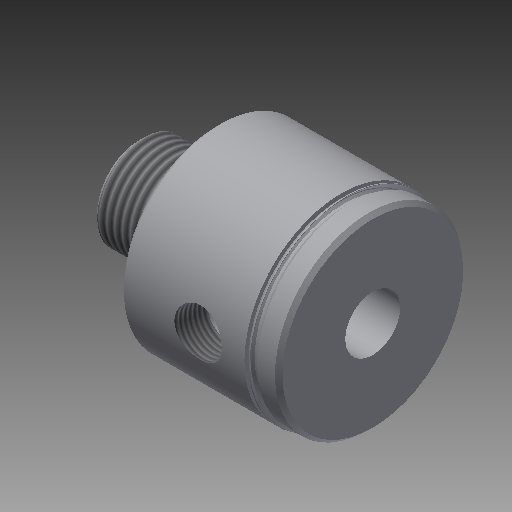
# Autodesk Inventor part: 17R000-0_rod_guide
Saved by Autodesk Inventor 2019.4 (Build 234330000, 330)
## iProperties
Category: PARTsolutions
Company: BIMBA
Created: 2020-02-18
Part Number: 17R000-0_rod_guide
Material: Generic
Catalog Web Link: www.cadenas.de
Description: Rod Guide-Original Line - Standard Air Cylinders
Vendor: BIMBA
Document SubType Name: Modeling
Designer: psadmin
Manufacturer: BIMBA
Mass: 37.006 g
Surface Area: 94.3607 cm^2
Volume: 37.006 cm^3
Density: 1 g/cm^3
Appearance: PSOLRGB-211-211-211
PSOL_IDENT_0: {$CADENAS_DATA\23d-libs\bimba\bimba_brand\bimba_imperial\bimba_full_line\original_line_cylinders\sta
PSOL_IDENT_1: ndard_air_cylinders\rod_guide.prj},251 {VTYP=3D},{NB=17R000-0_rod_guide},{LINA=17R000-0_rod_guide},{
PSOL_IDENT_2: NN=Rod Guide},{DATE=10.02.2020 11:55:59},{GEOMDATE=15.10.2019 12:06:01},{VERSION=},{LINEID=80},{WBVA
PSOL_IDENT_3: R=MNT,ACTING,NR,K,Q,T1,T2,T3,T4,MB,TRIM,CUSH,RODTRANS},{WBNUMERIC=MB,TRIM,CUSH,RODTRANS}  {NB=17R000
PSOL_IDENT_4: -0_rod_guide},{LINA=17R000-0_rod_guide},{KT=DUMMY},{PN=17R000},{BORE=1.50000000},{BOREPN=17},{MNT=},
PSOL_IDENT_5: {MNTALG='' , 'Front Nose' , 'BF' , 'Front Block' , 'BFT' , 'Front Trunnion' , 'A' , 'Adjustable Stro
PSOL_IDENT_6: ke','BR' , 'Rear Block'},{ACTING=R},{ACTINGALG= '' , 'Single Acting' , 'R' , 'Reverse/Double Acting'
PSOL_IDENT_7: },{NR=},{NRALG= '' , 'Without Non-rotating Rod' , 'NR' , 'With Non-rotating Rod' },{K=},{Q=},{QALG=
PSOL_IDENT_8: '' , 'Without Side Ported Rear Head' , 'Q' , 'With Side Ported Rear Head' },{T1=},{T2=},{T3=},{T4=}
PSOL_IDENT_9: ,{MB=0},{A1=1.8750},{A1N=1.3120},{A1P=1.8750},{A1B=2.3750},{A2=0.6250},{A2N=0.6250},{A2P=0.6250},{A3=
PSOL_IDENT_10: 1.0000},{A3N=0.1880},{A3P=1.0000},{A4=0.2525},{A4N=0.5000},{A4P=0.2525},{A5=0.0400},{A6=0.0000},{A6N=
PSOL_IDENT_11: 0.2500},{A6P=0.0000},{A7=0.2500},{A7N=0.6430},{A7P=0.2500},{A8=0.0300},{A8N=0.0300},{A8NR=0.0300},{D
PSOL_IDENT_12: 1=1.5565},{D1N=1.5565},{D1P=1.5565},{D1B=1.5800},{D2=1.5115},{D3=0.0000},{D3N=0.8120},{D3P=0.0000},{
PSOL_IDENT_13: D4=0.9690},{D4N=0.4730},{D4P=0.9690},{D4NR=0.4395},{D5=0.4420},{D5N=0.4420},{D5NR=0.4395},{C1=0.030}
PSOL_IDENT_14: ,{C2=0.0300},{C2N=0.0300},{C2P=0.0300},{C3=0.0000},{C3N=0.0000},{C3P=0.0000},{C4=0.0300},{C4N=0.0000
PSOL_IDENT_15: },{C4P=0.0300},{NDM=0.7500},{NDMN=0.7500},{NDMP=0.7500},{TAB=UNF},{D6=0.7475},{D6N=0.7475},{D6P=0.74
PSOL_IDENT_16: 75},{A9=0.0940},{A9N=0.0940},{A9P=0.0940},{D7=0.6535},{D7N=0.6535},{D7P=0.6535},{A10=0.0965},{A10N=0
PSOL_IDENT_17: .0965},{A10P=0.0965},{R1=0.0440},{R1N=0.0440},{R1P=0.0440},{D8=0.8120},{D9=0.7500},{D10=0.6880},{A11=
PSOL_IDENT_18: 0.8650},{A12=0.9590},{A13=1.1150},{A14=0.6250},{A14N=0.6250},{A14B=0.7190},{D11=0.2500},{D11N=0.2500
PSOL_IDENT_19: },{NDM2=0.4050},{NDM2N=0.4050},{NDM2DP=0.4200},{THREAD=0},{HEX=0.4375},{HEXN=0.4375},{S1=1.7500},{B1=
PSOL_IDENT_20: 0.1275},{B2=1.0050},{B22=0.0000},{DB=0.0000},{B3=0.6200},{B4=1.1300},{X1=0.1230},{X2=0.9975},{NDM3=0
PSOL_IDENT_21: .3125},{NDM4=0.2500},{NDM4DP=0.4950},{DD=1.7500},{CB=0.3750},{CBDP=0.2500},{PORT=1},{XT=1.0610},{XTX=
PSOL_IDENT_22: 1.0610},{XT1=0.5000},{XT2=0.3800},{NDMH=0.7500},{OD=1.5565},{ID=1.5115},{G=0.0000},{PNUT=0.5310},{TR
PSOL_IDENT_23: IM=0},{C11=0.3965},{C22=0.5625},{C33=0.3050},{C44=0.6250},{C55=0.8750},{CD1=0.2650},{CD2=0.1980},{CD
PSOL_IDENT_24: 3=0.1345},{CNDM3=0.2500},{CTAB3=UNS},{CUSH=0},{XX=1.13000},{LCD=0.0000},{RODTRANS=0.00000}
NN: Rod Guide
NT: Original Line - Standard Air Cylinders
NB: 17R000-0_rod_guide
NBSYN: $PN.-$RODTRANS._rod_guide
LINA: 17R000-0_rod_guide
BORE: 0
BOREPN: 17
MNT: Front Nose
MNTALG: '' , 'Front Nose' , 'BF' , 'Front Block' , 'BFT' , 'Front Trunnion' , 'A' , 'Adjustable Stroke','BR' , 'Rear Block'
ACTING: Reverse/Double Acting
NR: Without Non-rotating Rod
K: Standard
Q: Without Side Ported Rear Head
T1: without T1
T2: without T2
T3: without T3
T4: without T4
MB: 0
A1N: 1.312
A1P: 1.875
A1B: 2.375
A2N: 0.625
A2P: 0.625
A3N: 0.188
A3P: 1
A4N: 0.5
A4P: 0.2525
A5: 0.04
A6N: 0.25
A6P: 0
A7N: 0.643
A7P: 0.25
A8N: 0.03
A8NR: 0.03
D1N: 1.5565
D1P: 1.5565
D1B: 1.58
D2: 1.5115
D3N: 0.812
D3P: 0
D4N: 0.473
D4P: 0.969
D4NR: 0.4395
D5N: 0.442
D5NR: 0.4395
C1: 0.03
C2N: 0.03
C2P: 0.03
C3N: 0
C3P: 0
C4N: 0
C4P: 0.03
NDMN: 0.75
NDMP: 0.75
TAB: UNF
D6N: 0.7475
D6P: 0.7475
A9N: 0.094
A9P: 0.094
D7N: 0.6535
D7P: 0.6535
A10N: 0.0965
A10P: 0.0965
R1N: 0.044
R1P: 0.044
D8: 0.812
D9: 0.75
D10: 0.688
A11: 0.865
A12: 0.959
A13: 1.115
A14N: 0.625
A14B: 0.719
D11N: 0.25
NDM2N: 0.405
NDM2DP: 0.42
HEXN: 0.4375
S1: 1.75
B1: 0.1275
B2: 1.005
B22: 0
DB: 0
B3: 0.62
B4: 1.13
X1: 0.123
X2: 0.9975
NDM3: 0.3125
NDM4: 0.25
NDM4DP: 0.495
DD: 1.75
CB: 0.375
CBDP: 0.25
XTX: 1.061
XT1: 0.5
XT2: 0.38
NDMH: 0.75
TRIM: 0
C11: 0.3965
C22: 0.5625
C33: 0.305
C44: 0.625
C55: 0.875
CD1: 0.265
CD2: 0.198
CD3: 0.1345
CNDM3: 0.25
CTAB3: UNS
CUSH: 0
LCD: 0
RODTRANS: 0
SUPPLIER: BIMBA
ARTICLENO: 17R000-0_rod_guide
BOMINFO: 17R000-0_rod_guide
CREATOR: CADENAS GmbH
Title: 17R000-0_rod_guide
Author: Cadenas PARTsolutions
Comments: Original Line - Standard Air Cylinders
Autodesk Inventor part; units mm, degrees
ref_plane "YZ Plane" through (0, 0, 0) normal (1, 0, 0) x (0, 1, 0)
ref_plane "XZ Plane" through (0, 0, 0) normal (0, 1, 0) x (-1, 0, 0)
ref_plane "XY Plane" through (0, 0, 0) normal (0, 0, 1) x (1, 0, 0)
sketch "Sketch_2" plane through (0, 0, 0) normal (0, 0, 1) x (1, 0, 0)
  line L0 (15.875, 0) -> (0, 0)
  line L1 (0, 0) -> (0, 8.589)
  line L2 (0, 8.589) -> (0.936, 9.525)
  line L3 (0.936, 9.525) -> (9.31, 9.525)
  line L4 (9.31, 9.525) -> (10.2623, 8.6108)
  arc A0 (10.2623, 8.6108) -> (11.0363, 8.2995) centre (11.0363, 9.417) ccw
  line L5 (11.0363, 8.2995) -> (12.3698, 8.2995)
  arc A1 (12.3698, 8.2995) -> (13.4874, 9.417) centre (12.3698, 9.4171) ccw
  line L6 (13.4874, 9.417) -> (13.4874, 9.4932)
  line L7 (13.4874, 9.4932) -> (15.875, 9.4932)
  line L8 (15.875, 9.4932) -> (15.875, 0)
  line L9 (15.875, 0) -> (0, 0)
  constraints: 20 end point, 4 point on circle, 2 centre point
revolve "Revolution1" add sketch "Sketch_2" angle 360 about axis through (15.875, 0, 0) along (1, 0, 0)
thread "Thread1" size "3/4-16 UNF" class "2A" standard "ANSI Unified Screw Threads" full length
sketch "Sketch_3" plane through (0, 0, 0) normal (0, 0, 1) x (1, 0, 0)
  line L0 (47.625, 0) -> (15.875, 0)
  line L1 (15.875, 0) -> (15.875, 19.0055)
  line L2 (15.875, 19.0055) -> (16.637, 19.7675)
  line L3 (16.637, 19.7675) -> (41.2115, 19.7675)
  line L4 (41.2115, 19.7675) -> (41.2115, 18.1801)
  line L5 (41.2115, 18.1801) -> (42.2275, 18.1801)
  line L6 (42.2275, 18.1801) -> (43.2435, 19.196)
  line L7 (43.2435, 19.196) -> (46.863, 19.196)
  line L8 (46.863, 19.196) -> (47.625, 18.434)
  line L9 (47.625, 18.434) -> (47.625, 0)
  line L10 (47.625, 0) -> (15.875, 0)
  constraints: 22 end point
revolve "Revolution2" add sketch "Sketch_3" angle 360 about axis through (47.625, 0, 0) along (1, 0, 0)
sketch "Sketch3" plane through (0, 0, 0) normal (-1, 0, 0) x (0, 0, 1)
  point P0 (0, 0)
hole "Hole1" at (0, 0, 0) direction (1, 0, 0) diameter 11.2268 depth 47.625 countersink diameter 12.7508 countersink angle 90
sketch "Sketch_40" plane through (0, 0, 0) normal (0, 1, 0) x (-1, 0, 0)
  line L0 (-31.75, 19.7675) -> (-31.75, 0)
  line L1 (-31.75, 0) -> (-34.925, 0)
  line L2 (-34.925, 0) -> (-34.925, 7.7681)
  line L3 (-34.925, 7.7681) -> (-36.2564, 9.0996)
  line L4 (-36.2564, 9.0996) -> (-36.5895, 19.7675)
  line L5 (-36.5895, 19.7675) -> (-31.75, 19.7675)
  line L6 (-31.75, 19.7675) -> (-31.75, 0)
  constraints: 14 end point
revolve "Revolution3" cut sketch "Sketch_40" angle 360 about axis through (31.75, 0, 19.7675) along (0, 0, 1)
thread "Thread2" size "1/8" designation "1/8 - 27 NPT" standard "NPT" length 6.4039
sketch "Sketch_47" plane through (0, 0, 0) normal (0, 0, 1) x (1, 0, 0)
  line L0 (42.2275, 0) -> (41.2115, 0)
  line L1 (41.2115, 18.8883) -> (41.2115, 17.9261)
  line L2 (41.2115, 17.9261) -> (42.2275, 17.9261)
  line L3 (42.2275, 17.9261) -> (42.2275, 18.1801)
  line L4 (42.2275, 18.1801) -> (41.7195, 18.1801)
  line L5 (41.7195, 18.1801) -> (41.3449, 18.5547)
  arc A0 (41.3449, 18.7343) -> (41.3449, 18.5547) centre (41.4347, 18.6445) ccw
  line L6 (41.3449, 18.7343) -> (42.294, 19.6834)
  line L7 (42.294, 19.6834) -> (42.294, 19.7675)
  line L8 (42.294, 19.7675) -> (42.0908, 19.7675)
  line L9 (42.0908, 19.7675) -> (41.2115, 18.8883)
  constraints: 20 end point, 2 point on circle, 1 centre point
revolve "Revolution4" add sketch "Sketch_47" angle 360 about axis through (42.2275, 0, 0) along (1, 0, 0)
ref_plane "dp1_XY" through (15.875, 9.4932, 0) normal (0, 0, 1) x (1, 0, 0)
ref_plane "dp1_YZ" through (15.875, 9.4932, 0) normal (1, 0, 0) x (0, 1, 0)
ref_plane "dp1_ZX" through (15.875, 9.4932, 0) normal (0, 1, 0) x (0, 0, 1)
ref_plane "dp2_XY" through (15.875, -9.4932, 0) normal (0, 0, 1) x (1, 0, 0)
ref_plane "dp2_YZ" through (15.875, -9.4932, 0) normal (1, 0, 0) x (0, 1, 0)
ref_plane "dp2_ZX" through (15.875, -9.4932, 0) normal (0, 1, 0) x (0, 0, 1)
ref_plane "hh_XY" through (0, 9.525, 0) normal (0, 0, 1) x (1, 0, 0)
ref_plane "hh_YZ" through (0, 9.525, 0) normal (1, 0, 0) x (0, 1, 0)
ref_plane "hh_ZX" through (0, 9.525, 0) normal (0, 1, 0) x (0, 0, 1)
ref_plane "port_XY" through (31.75, 0, 0) normal (0, 0, 1) x (1, 0, 0)
ref_plane "port_YZ" through (31.75, 0, 0) normal (1, 0, 0) x (0, 1, 0)
ref_plane "port_ZX" through (31.75, 0, 0) normal (0, 1, 0) x (0, 0, 1)
ref_plane "rod_guide_XY" through (0, 0, 0) normal (1, 0, 0) x (0, 0, -1)
ref_plane "rod_guide_YZ" through (0, 0, 0) normal (0, 0, -1) x (0, 1, 0)
ref_plane "rod_guide_ZX" through (0, 0, 0) normal (0, 1, 0) x (1, 0, 0)
ref_plane "s1_XY" through (13.4874, 0, 0) normal (0, 0, 1) x (1, 0, 0)
ref_plane "s1_YZ" through (13.4874, 0, 0) normal (1, 0, 0) x (0, 1, 0)
ref_plane "s1_ZX" through (13.4874, 0, 0) normal (0, 1, 0) x (0, 0, 1)
ref_plane "s2_XY" through (15.875, 0, 0) normal (0, 0, 1) x (1, 0, 0)
ref_plane "s2_YZ" through (15.875, 0, 0) normal (1, 0, 0) x (0, 1, 0)
ref_plane "s2_ZX" through (15.875, 0, 0) normal (0, 1, 0) x (0, 0, 1)
ref_plane "t1_XY" through (15.875, 0, 0) normal (1, 0, 0) x (0, 0, -1)
ref_plane "t1_YZ" through (15.875, 0, 0) normal (0, 0, -1) x (0, 1, 0)
ref_plane "t1_ZX" through (15.875, 0, 0) normal (0, 1, 0) x (1, 0, 0)
ref_plane "t111_XY" through (15.875, 0, 0) normal (1, 0, 0) x (0, 0, -1)
ref_plane "t111_YZ" through (15.875, 0, 0) normal (0, 0, -1) x (0, 1, 0)
ref_plane "t111_ZX" through (15.875, 0, 0) normal (0, 1, 0) x (1, 0, 0)
ref_plane "to_foot_bracket_XY" through (15.875, 0, 0) normal (1, 0, 0) x (0, 0, -1)
ref_plane "to_foot_bracket_YZ" through (15.875, 0, 0) normal (0, 0, -1) x (0, 1, 0)
ref_plane "to_foot_bracket_ZX" through (15.875, 0, 0) normal (0, 1, 0) x (1, 0, 0)
ref_plane "to_nut_XY" through (13.4874, 0, 0) normal (1, 0, 0) x (0, 0, -1)
ref_plane "to_nut_YZ" through (13.4874, 0, 0) normal (0, 0, -1) x (0, 1, 0)
ref_plane "to_nut_ZX" through (13.4874, 0, 0) normal (0, 1, 0) x (1, 0, 0)
ref_plane "to_rod_XY" through (0, 0, 0) normal (1, 0, 0) x (0, 0, -1)
ref_plane "to_rod_YZ" through (0, 0, 0) normal (0, 0, -1) x (0, 1, 0)
ref_plane "to_rod_ZX" through (0, 0, 0) normal (0, 1, 0) x (1, 0, 0)
ref_plane "to_screw_XY" through (31.75, 14.2875, -10.0711) normal (0, 1, 0) x (1, 0, 0)
ref_plane "to_screw_YZ" through (31.75, 14.2875, -10.0711) normal (1, 0, 0) x (0, 0, -1)
ref_plane "to_screw_ZX" through (31.75, 14.2875, -10.0711) normal (0, 0, -1) x (0, 1, 0)
ref_plane "to_trunnion_brackets_XY" through (26.9494, 0, 0) normal (0, 1, 0) x (1, 0, 0)
ref_plane "to_trunnion_brackets_YZ" through (26.9494, 0, 0) normal (1, 0, 0) x (0, 0, -1)
ref_plane "to_trunnion_brackets_ZX" through (26.9494, 0, 0) normal (0, 0, -1) x (0, 1, 0)
ref_plane "to_trunnion_brackets1_XY" through (26.9494, 22.225, 0) normal (0, 1, 0) x (1, 0, 0)
ref_plane "to_trunnion_brackets1_YZ" through (26.9494, 22.225, 0) normal (1, 0, 0) x (0, 0, -1)
ref_plane "to_trunnion_brackets1_ZX" through (26.9494, 22.225, 0) normal (0, 0, -1) x (0, 1, 0)
ref_plane "to_trunnion_brackets2_XY" through (26.9494, -22.225, 0) normal (0, 1, 0) x (1, 0, 0)
ref_plane "to_trunnion_brackets2_YZ" through (26.9494, -22.225, 0) normal (1, 0, 0) x (0, 0, -1)
ref_plane "to_trunnion_brackets2_ZX" through (26.9494, -22.225, 0) normal (0, 0, -1) x (0, 1, 0)
ref_plane "to_tube_XY" through (42.2275, 0, 0) normal (1, 0, 0) x (0, 0, -1)
ref_plane "to_tube_YZ" through (42.2275, 0, 0) normal (0, 0, -1) x (0, 1, 0)
ref_plane "to_tube_ZX" through (42.2275, 0, 0) normal (0, 1, 0) x (1, 0, 0)
body "Solid1"
